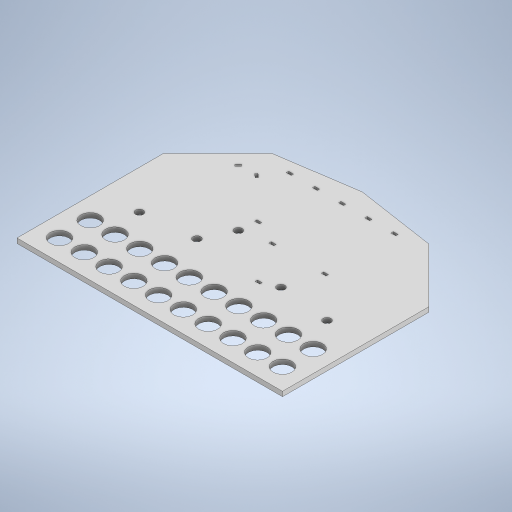
# Autodesk Inventor part: ChannelInsert
Saved by Autodesk Inventor 2023 (Build 270158000, 158)
## iProperties
Created: 2023-05-02
Part Number: ChannelInsert
Material: Generic
Document SubType Name: Modeling
Designer: 1roweste
Density: 1 g/cm^3
Appearance: Default
Author: 1roweste
Autodesk Inventor part; units mm, degrees
ref_plane "YZ Plane" through (0, 0, 0) normal (1, 0, 0) x (0, 1, 0)
ref_plane "XZ Plane" through (0, 0, 0) normal (0, 1, 0) x (-1, 0, 0)
ref_plane "XY Plane" through (0, 0, 0) normal (0, 0, 1) x (1, 0, 0)
sketch "Sketch1" plane through (0, 0, 0) normal (0, 1, 0) x (-1, 0, 0)
  line L0 (0, 2) -> (-5.5, 2)
  line L1 (-5.5, -125.4) -> (-5.5, 2)
  line L2 (0, -125.4) -> (-5.5, -125.4)
  line L3 (0, -125.4) -> (0, -123.4)
  line L4 (0, -123.4) -> (65.1, -123.4)
  line L5 (65.1, -122.571573) -> (65.1, -123.4)
  line L6 (65.1, -122.571573) -> (88.858788, -98.812785)
  line L7 (88.858788, -98.812785) -> (84.969701, -94.923698)
  line L8 (84.969701, -94.923698) -> (61.993398, -117.9)
  line L9 (0, -117.9) -> (61.993398, -117.9)
  line L10 (0, -117.9) -> (0, -5.5)
  line L11 (0, -5.5) -> (61.993398, -5.5)
  line L12 (84.969701, -28.476302) -> (61.993398, -5.5)
  line L13 (88.858788, -24.587215) -> (84.969701, -28.476302)
  line L14 (65.1, -0.828427) -> (88.858788, -24.587215)
  line L15 (65.1, 0) -> (65.1, -0.828427)
  line L16 (0, 0) -> (65.1, 0)
  line L17 (0, 0) -> (0, 2)
  line L18 (84.969701, -28.476302) -> (84.969701, -94.923698)
  line L19 (84.616147, -94.570144) -> (61.786292, -117.4)
  line L20 (61.786292, -117.4) -> (0.5, -117.4)
  line L21 (0.5, -117.4) -> (0.5, -6)
  line L22 (0.5, -6) -> (61.786292, -6)
  line L23 (61.786292, -6) -> (84.616147, -28.829856)
  point P0 (94.5, -125.4)
  dimension "d0" = 0.5
  constraints: 48 end point, 1 vertical, 4 other
  measures "d0" distance between parallel lines of L9 L20
extrude "Extrusion1" add sketch "Sketch1" along normal blind 2 contours L18 L8 L9 L10 L11 L12
sketch "Sketch2" plane through (0, 2, 0) normal (0, 1, 0) x (1, 0, 0)
  line L0 (-61.993398, 117.9) -> (-84.969701, 94.923698)
  line L1 (-84.969701, 94.923698) -> (-84.969701, 28.476302)
  line L2 (-84.969701, 28.476302) -> (-61.993398, 5.5)
  line L3 (-61.993398, 5.5) -> (0, 5.5)
  line L4 (0, 5.5) -> (0, 117.9)
  line L5 (0, 117.9) -> (-61.993398, 117.9)
  line L6 (-84.969701, 61.7) -> (-89.969701, 61.7)
  line L7 (-89.969701, 61.7) -> (-84.969701, 28.476302)
  line L8 (-89.969701, 61.7) -> (-84.969701, 94.923698)
  point P0 (0, 0)
  dimension "d3" = 5
  constraints: 6 end point, 1 horizontal, 1 midpoint
  measures "d3" distance of L6.start L6.end
extrude "Extrusion2" add sketch "Sketch2" against normal blind 1 contours L1 L6 L8 | L1 L7 L6
sketch "Sketch3" plane through (0, 2, 0) normal (0, 1, 0) x (1, 0, 0)
  line L0 (-84.969701, 94.923698) -> (-84.969701, 28.476302)
  line L1 (-81.969701, 94.923698) -> (-81.969701, 28.476302)
  line L2 (-80.969701, 62.7) -> (-81.969701, 62.7)
  line L3 (-81.969701, 62.7) -> (-81.969701, 60.7)
  line L4 (-81.969701, 60.7) -> (-80.969701, 60.7)
  line L5 (-80.969701, 60.7) -> (-80.969701, 62.7)
  line L6 (-80.969701, 51.625333) -> (-81.969701, 51.625333)
  line L7 (-81.969701, 51.625333) -> (-81.969701, 49.625333)
  line L8 (-81.969701, 49.625333) -> (-80.969701, 49.625333)
  line L9 (-80.969701, 49.625333) -> (-80.969701, 51.625333)
  line L10 (-80.969701, 40.550667) -> (-81.969701, 40.550667)
  line L11 (-81.969701, 40.550667) -> (-81.969701, 38.550667)
  line L12 (-81.969701, 38.550667) -> (-80.969701, 38.550667)
  line L13 (-80.969701, 38.550667) -> (-80.969701, 40.550667)
  line L14 (-80.969701, 73.774667) -> (-81.969701, 73.774667)
  line L15 (-81.969701, 73.774667) -> (-81.969701, 71.774667)
  line L16 (-81.969701, 71.774667) -> (-80.969701, 71.774667)
  line L17 (-80.969701, 71.774667) -> (-80.969701, 73.774667)
  line L18 (-80.969701, 62.7) -> (-81.969701, 62.7)
  line L19 (-81.969701, 62.7) -> (-81.969701, 60.7)
  line L20 (-81.969701, 60.7) -> (-80.969701, 60.7)
  line L21 (-80.969701, 60.7) -> (-80.969701, 62.7)
  line L22 (-80.969701, 51.625333) -> (-81.969701, 51.625333)
  line L23 (-81.969701, 51.625333) -> (-81.969701, 49.625333)
  line L24 (-81.969701, 49.625333) -> (-80.969701, 49.625333)
  line L25 (-80.969701, 49.625333) -> (-80.969701, 51.625333)
  line L26 (-80.969701, 84.849333) -> (-81.969701, 84.849333)
  line L27 (-81.969701, 84.849333) -> (-81.969701, 82.849333)
  line L28 (-81.969701, 82.849333) -> (-80.969701, 82.849333)
  line L29 (-80.969701, 82.849333) -> (-80.969701, 84.849333)
  line L30 (-80.969701, 73.774667) -> (-81.969701, 73.774667)
  line L31 (-81.969701, 73.774667) -> (-81.969701, 71.774667)
  line L32 (-81.969701, 71.774667) -> (-80.969701, 71.774667)
  line L33 (-80.969701, 71.774667) -> (-80.969701, 73.774667)
  line L34 (-80.969701, 62.7) -> (-81.969701, 62.7)
  line L35 (-81.969701, 62.7) -> (-81.969701, 60.7)
  line L36 (-81.969701, 60.7) -> (-80.969701, 60.7)
  line L37 (-80.969701, 60.7) -> (-80.969701, 62.7)
  point P0 (0, 0)
  point P1 (-81.969701, 61.7)
  point P2 (-81.969701, 61.7)
  point P3 (-80.969701, 61.7)
  point P4 (-81.969701, 50.625333)
  point P5 (-80.969701, 50.625333)
  point P6 (-81.969701, 50.625333)
  point P7 (-81.969701, 39.550667)
  point P8 (-80.969701, 39.550667)
  point P9 (-81.969701, 39.550667)
  point P10 (-81.969701, 72.774667)
  point P11 (-80.969701, 72.774667)
  point P12 (-81.969701, 72.774667)
  point P13 (-81.969701, 61.7)
  point P14 (-80.969701, 61.7)
  point P15 (-81.969701, 61.7)
  point P16 (-81.969701, 50.625333)
  point P17 (-80.969701, 50.625333)
  point P18 (-81.969701, 50.625333)
  point P19 (-81.969701, 83.849333)
  point P20 (-80.969701, 83.849333)
  point P21 (-81.969701, 83.849333)
  point P22 (-81.969701, 72.774667)
  point P23 (-80.969701, 72.774667)
  point P24 (-81.969701, 72.774667)
  point P25 (-81.969701, 61.7)
  point P26 (-80.969701, 61.7)
  point P27 (-81.969701, 61.7)
  dimension "d6" = 3
  dimension "d7" = 1
  dimension "d8" = 2
  dimension "d9" = 0
  dimension "d10" = 0
  dimension "d13" = 11.07467
  dimension "d16" = 11.07467
  constraints: 76 end point, 3 midpoint, 3 parallel, 2 vertical, 1 horizontal, 1 perpendicular, 88 other
  measures "d6" distance between parallel lines of L0 L1
  measures "d7" distance of L4.end L3.end
  measures "d8" distance of L3.end L2.end
  measures "d9" distance from line of L1 point (-81.97, 61.7)
  measures "d10" vertical distance of point (-81.97, 61.7) point (-80.97, 61.7)
  measures "d13" distance of L2.start L6.start
  measures "d16" distance of L2.start L14.start
extrude "Extrusion3" cut sketch "Sketch3" against normal blind 2
sketch "Sketch4" plane through (0, 2, 0) normal (0, 1, 0) x (1, 0, 0)
  line L0 (0, -2) -> (5.5, -2)
  line L1 (5.5, 125.4) -> (5.5, -2)
  line L2 (0, 125.4) -> (5.5, 125.4)
  line L3 (0, 125.4) -> (0, 123.4)
  line L4 (0, 123.4) -> (-65.1, 123.4)
  line L5 (-65.1, 122.571573) -> (-65.1, 123.4)
  line L6 (-65.1, 122.571573) -> (-88.858788, 98.812785)
  line L7 (-88.858788, 98.812785) -> (-84.969701, 94.923698)
  line L8 (-84.969701, 94.923698) -> (-61.993398, 117.9)
  line L9 (0, 117.9) -> (-61.993398, 117.9)
  line L10 (0, 117.9) -> (0, 5.5)
  line L11 (0, 5.5) -> (-61.993398, 5.5)
  line L12 (-88.858788, 24.587215) -> (-84.969701, 28.476302)
  line L13 (-65.1, 0.828427) -> (-88.858788, 24.587215)
  line L14 (-65.1, 0) -> (-65.1, 0.828427)
  line L15 (0, 0) -> (-65.1, 0)
  line L16 (0, 0) -> (0, -2)
  circle A0 centre (-79.431925, 19.770487) radius 1
  line L17 (-55.8, 5.5) -> (-53.8, 5.5)
  circle A1 centre (-54.8, 3.25) radius 1
  circle A2 centre (2.25, 8.3) radius 1
  line L18 (0, 7.3) -> (0, 9.3)
  circle A3 centre (2.25, 43.9) radius 1
  line L19 (0, 42.9) -> (0, 44.9)
  circle A4 centre (2.25, 79.5) radius 1
  line L20 (0, 78.5) -> (0, 80.5)
  circle A5 centre (2.25, 115.1) radius 1
  line L21 (0, 114.1) -> (0, 116.1)
  circle A6 centre (-54.8, 120.15) radius 1
  line L22 (-53.8, 117.9) -> (-55.8, 117.9)
  circle A7 centre (-79.487689, 103.587689) radius 1
  line L23 (-77.189592, 102.703806) -> (-78.603806, 101.289592)
  line L24 (-81.969701, 60.7) -> (-81.969701, 62.7)
  line L25 (-81.969701, 62.7) -> (-80.969701, 62.7)
  line L26 (-80.969701, 62.7) -> (-80.969701, 60.7)
  line L27 (-80.969701, 60.7) -> (-81.969701, 60.7)
  line L28 (-81.969701, 49.625333) -> (-81.969701, 51.625333)
  line L29 (-81.969701, 51.625333) -> (-80.969701, 51.625333)
  line L30 (-80.969701, 51.625333) -> (-80.969701, 49.625333)
  line L31 (-80.969701, 49.625333) -> (-81.969701, 49.625333)
  line L32 (-81.969701, 71.774667) -> (-81.969701, 73.774667)
  line L33 (-81.969701, 73.774667) -> (-80.969701, 73.774667)
  line L34 (-80.969701, 73.774667) -> (-80.969701, 71.774667)
  line L35 (-80.969701, 71.774667) -> (-81.969701, 71.774667)
  line L36 (-81.969701, 38.550667) -> (-81.969701, 40.550667)
  line L37 (-81.969701, 40.550667) -> (-80.969701, 40.550667)
  line L38 (-80.969701, 40.550667) -> (-80.969701, 38.550667)
  line L39 (-80.969701, 38.550667) -> (-81.969701, 38.550667)
  line L40 (-81.969701, 82.849333) -> (-81.969701, 84.849333)
  line L41 (-81.969701, 84.849333) -> (-80.969701, 84.849333)
  line L42 (-80.969701, 84.849333) -> (-80.969701, 82.849333)
  line L43 (-80.969701, 82.849333) -> (-81.969701, 82.849333)
  line L44 (-61.993398, 117.9) -> (-84.969701, 94.923698)
  line L45 (-84.969701, 94.923698) -> (-89.969701, 61.7)
  line L46 (-89.969701, 61.7) -> (-84.969701, 28.476302)
  line L47 (-84.969701, 28.476302) -> (-61.993398, 5.5)
  line L48 (-61.993398, 5.5) -> (0, 5.5)
  line L49 (0, 5.5) -> (0, 117.9)
  line L50 (0, 117.9) -> (-61.993398, 117.9)
  line L51 (0, 117.9) -> (-61.993398, 117.9)
  line L52 (-89.969701, 61.7) -> (-84.969701, 94.923698)
  line L53 (-84.969701, 94.923698) -> (-84.969701, 28.476302)
  line L54 (-84.969701, 94.923698) -> (-84.969701, 28.476302)
  circle A8 centre (-42.48485, 61.7) radius 0.5
  line L55 (-84.969701, 28.476302) -> (-84.969701, 94.923698)
  line L56 (-84.969701, 61.7) -> (0, 61.7)
  circle A9 centre (-42.48485, 61.7) radius 0.5
  line L57 (-81.969701, 72.774667) -> (-34.999701, 72.774667)
  line L58 (-81.969701, 72.774667) -> (-34.999701, 72.774667) construction
  line L59 (-81.969701, 83.849333) -> (-51.969701, 83.849333)
  line L60 (-81.969701, 83.849333) -> (-51.969701, 83.849333) construction
  line L61 (-81.969701, 61.7) -> (-51.969701, 61.7)
  line L62 (-81.969701, 61.7) -> (-51.969701, 61.7) construction
  line L63 (-81.969701, 51.625333) -> (-81.969701, 49.625333)
  line L64 (-81.969701, 50.625333) -> (-56.969701, 50.625333)
  line L65 (-81.969701, 50.625333) -> (-56.969701, 50.625333) construction
  line L66 (-79.431925, 19.770487) -> (-61.754255, 37.448157)
  line L67 (-79.431925, 19.770487) -> (-54.431925, 19.770487) construction
  line L68 (-80.969701, 38.550667) -> (-80.969701, 40.550667)
  line L69 (-80.969701, 39.550667) -> (-59.64794, 21.659585)
  line L70 (-80.969701, 39.550667) -> (-53.136118, 39.550667) construction
  line L71 (-73.317867, 34.435423) -> (-74.603442, 32.903334)
  line L72 (-74.603442, 32.903334) -> (-73.837398, 32.260547)
  line L73 (-73.837398, 32.260547) -> (-72.551823, 33.792636)
  line L74 (-72.551823, 33.792636) -> (-73.317867, 34.435423)
  line L75 (-73.19461, 33.026591) -> (-73.19461, 21.984973)
  line L76 (-73.19461, 33.026591) -> (-62.152992, 33.026591) construction
  line L77 (-74.608824, 26.007802) -> (-73.19461, 24.593589)
  line L78 (-74.608824, 26.007802) -> (-73.901717, 26.714909)
  line L79 (-73.901717, 26.714909) -> (-72.487503, 25.300695)
  line L80 (-72.487503, 25.300695) -> (-73.19461, 24.593589)
  line L81 (-51.469701, 84.849333) -> (-52.469701, 84.849333)
  line L82 (-52.469701, 84.849333) -> (-52.469701, 82.849333)
  line L83 (-52.469701, 82.849333) -> (-51.469701, 82.849333)
  line L84 (-51.469701, 82.849333) -> (-51.469701, 84.849333)
  line L85 (-34.499701, 73.774667) -> (-35.499701, 73.774667)
  line L86 (-35.499701, 73.774667) -> (-35.499701, 71.774667)
  line L87 (-35.499701, 71.774667) -> (-34.499701, 71.774667)
  line L88 (-34.499701, 71.774667) -> (-34.499701, 73.774667)
  line L89 (-51.469701, 62.7) -> (-52.469701, 62.7)
  line L90 (-52.469701, 62.7) -> (-52.469701, 60.7)
  line L91 (-52.469701, 60.7) -> (-51.469701, 60.7)
  line L92 (-51.469701, 60.7) -> (-51.469701, 62.7)
  line L93 (-56.469701, 51.625333) -> (-57.469701, 51.625333)
  line L94 (-57.469701, 51.625333) -> (-57.469701, 49.625333)
  line L95 (-57.469701, 49.625333) -> (-56.469701, 49.625333)
  line L96 (-56.469701, 49.625333) -> (-56.469701, 51.625333)
  line L97 (-77.847905, 21.354507) -> (-49.563634, 49.638778)
  circle A10 centre (-49.563634, 49.638778) radius 1.65
  line L98 (2.25, 115.1) -> (-35.337705, 101.419194)
  line L99 (2.25, 115.1) -> (42.25, 115.1) construction
  line L100 (2.25, 79.5) -> (-37.75, 79.5)
  line L101 (2.25, 43.9) -> (-37.75, 43.9)
  line L102 (2.25, 8.3) -> (-35.337705, 21.980806)
  line L103 (2.25, 8.3) -> (42.25, 8.3) construction
  circle A11 centre (-35.337705, 101.419194) radius 1.65
  circle A12 centre (-37.75, 79.5) radius 1.65
  circle A13 centre (-37.75, 43.9) radius 1.65
  circle A14 centre (-35.337705, 21.980806) radius 1.65
  point P0 (0, 0)
  point P1 (8.532457, 50.928666)
  point P2 (-73.960655, 33.669379)
  point P3 (-73.901717, 25.300695)
  point P4 (-73.19461, 26.007802)
  point P5 (-52.469701, 83.849333)
  point P6 (-51.969701, 84.849333)
  point P7 (-35.499701, 72.774667)
  point P8 (-34.999701, 73.774667)
  point P9 (-52.469701, 61.7)
  point P10 (-51.969701, 62.7)
  point P11 (-56.969701, 51.625333)
  dimension "d25" = 46.97
  dimension "d27" = 30
  dimension "d28" = 0
  dimension "d29" = 30
  dimension "d30" = 0
  dimension "d31" = 25
  dimension "d32" = 0
  dimension "d33" = 25
  dimension "d34" = 45
  dimension "d35" = 40
  dimension "d38" = 2
  dimension "d39" = 0
  dimension "d40" = 1
  dimension "d41" = 90
  dimension "d42" = 2
  dimension "d43" = 0
  dimension "d44" = 1
  dimension "d45" = 0
  dimension "d46" = 1
  dimension "d47" = 2
  dimension "d48" = 0
  dimension "d49" = 0
  dimension "d50" = 1
  dimension "d51" = 2
  dimension "d52" = 0
  dimension "d53" = 0
  dimension "d54" = 1
  dimension "d55" = 2
  dimension "d56" = 0
  dimension "d57" = 0
  dimension "d58" = 1
  dimension "d59" = 2
  dimension "d60" = 0
  dimension "d64" = 40
  dimension "d65" = 3.3
  dimension "d66" = 40
  dimension "d67" = 160
  dimension "d68" = 40
  dimension "d69" = 40
  dimension "d70" = 160
  dimension "d71" = 3.3
  dimension "d72" = 3.3
  dimension "d73" = 3.3
  dimension "d74" = 3.3
  constraints: 144 end point, 19 midpoint, 17 horizontal, 15 centre point, 11 parallel, 11 perpendicular, 9 equal length, 5 coincident, 4 point on line, 1 collinear, 1 vertical
  measures "d25" distance of L57.start L57.end
  measures "d27" distance of L59.start L59.end
  measures "d28" distance between parallel lines of L59 L60
  measures "d29" distance of L61.start L61.end
  measures "d30" distance between parallel lines of L61 L62
  measures "d31" distance of L64.start L64.end
  measures "d32" distance between parallel lines of L64 L65
  measures "d33" distance of L66.start L66.end
  measures "d34" angle of L67 L66
  measures "d35" angle of L69 L70
  measures "d38" distance of L71.start L71.end
  measures "d39" distance from line of L69 point (-73.961, 33.669)
  measures "d40" distance of L71.end L72.end
  measures "d41" angle of L75 L76
  measures "d42" distance of L77.start L77.end
  measures "d43" distance from line of L66 point (-73.902, 25.301)
  measures "d44" distance of L77.start L78.end
  measures "d45" distance from line of point (-73.195, 26.008) L75
  measures "d46" distance of L83.end L82.end
  measures "d47" distance of L82.end L81.end
  measures "d48" vertical distance of L59.end point (-52.47, 83.849)
  measures "d49" horizontal distance of L59.end point (-51.97, 84.849)
  measures "d50" distance of L87.end L86.end
  measures "d51" distance of L86.end L85.end
  measures "d52" vertical distance of L57.end point (-35.5, 72.775)
  measures "d53" horizontal distance of L57.end point (-35, 73.775)
  measures "d54" distance of L91.end L90.end
  measures "d55" distance of L90.end L89.end
  measures "d56" distance from line of L56 point (-52.47, 61.7)
  measures "d57" horizontal distance of L61.end point (-51.97, 62.7)
  measures "d58" distance of L95.end L94.end
  measures "d59" distance of L94.end L93.end
  measures "d60" horizontal distance of L65.end point (-56.97, 51.625)
  measures "d64" distance of L97.start L97.end
  measures "d65" diameter of A10
  measures "d66" distance of L98.start L98.end
  measures "d67" angle of L98 L99
  measures "d68" distance of L100.start L100.end
  measures "d69" distance of L102.start L102.end
  measures "d70" angle of L103 L102
  measures "d71" diameter of A11
  measures "d72" diameter of A12
  measures "d73" diameter of A13
  measures "d74" diameter of A14
extrude "Extrusion4" cut sketch "Sketch4" against normal blind 10 contours L90 L89 L92 L56 | L56 L92 L91 L90 | L77 L78 L79 L66 | L73 L72 L71 L69 | L69 L71 L74 L73 | L66 L75 L77 | L79 L80 L75 | L84 L83 L82 L81 | L88 L87 L86 L85 | L96 L95 L94 L93 | A10 | A11 | A12 | A13 | A14
sketch "Sketch5" plane through (0, 2, 0) normal (0, 1, 0) x (1, 0, 0)
  circle A0 centre (-9, 108.9) radius 4
  line L0 (0, 117.9) -> (-61.993398, 117.9)
  line L1 (0, 5.5) -> (0, 117.9)
  circle A1 centre (-9, 14.5) radius 4
  line L2 (-61.993398, 5.5) -> (0, 5.5)
  line L3 (-9, 108.9) -> (0, 108.9)
  line L4 (-9, 14.5) -> (0, 14.5)
  point P0 (0, 0)
  dimension "d75" = 8
  dimension "d76" = 9
  dimension "d77" = 9
  dimension "d80" = 8
  dimension "d81" = 9
  dimension "d82" = 9
  constraints: 4 end point, 2 centre point, 2 point on line, 1 horizontal, 1 perpendicular
  measures "d75" diameter of A0
  measures "d76" distance from line of L0 L3.start
  measures "d77" distance from line of L1 L3.start
  measures "d80" diameter of A1
  measures "d81" distance from line of L2 L4.start
  measures "d82" distance from line of L1 L4.start
extrude "Extrusion5" cut sketch "Sketch5" against normal blind 10 contours A0
pattern_linear "Rectangular Pattern1" count 10 spacing 10.488889 along (0, 0, 1) count 2 spacing 13 along (-1, 0, 0) of "Extrusion5"
body "Solid1"
